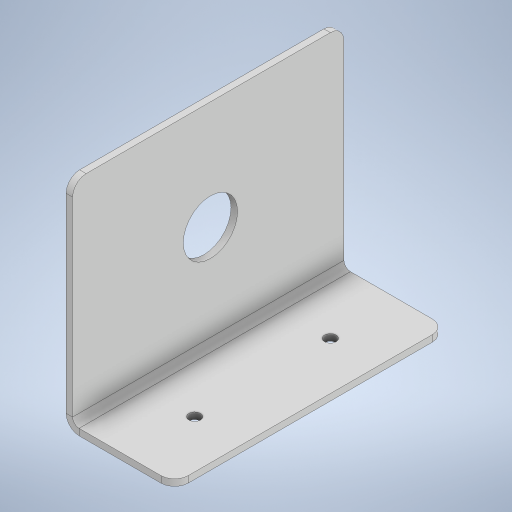
# Autodesk Inventor part: Bracket
Saved by Autodesk Inventor 2023 (Build 270158030, 158C)
## iProperties
Created: 2022-10-06
Part Number: Bracket
Material: Generic
Document SubType Name: Sheet Metal
Designer: cjj5381
Density: 1 g/cm^3
Sheet Metal Rule: Default
Appearance: Default
Author: cjj5381
Autodesk Inventor part; units mm, degrees
ref_plane "YZ Plane" through (0, 0, 0) normal (1, 0, 0) x (0, 1, 0)
ref_plane "XZ Plane" through (0, 0, 0) normal (0, 1, 0) x (-1, 0, 0)
ref_plane "XY Plane" through (0, 0, 0) normal (0, 0, 1) x (1, 0, 0)
sketch "Sketch1" plane through (0, 0, 0) normal (0, 1, 0) x (-1, 0, 0)
  line L0 (-25.4, 63.5) -> (25.4, 63.5)
  line L1 (25.4, 63.5) -> (25.4, -63.5)
  line L2 (25.4, -63.5) -> (-25.4, -63.5)
  line L3 (-25.4, -63.5) -> (-25.4, 63.5)
  line L4 (-25.4, 63.5) -> (25.4, -63.5) construction
  line L5 (25.4, 63.5) -> (-25.4, -63.5) construction
  point P0 (0, 0)
  dimension "d0" = 50.8
  dimension "d1" = 127
  measures "d0" distance of L1.end L2.end
  measures "d1" distance of L0.end L1.end
extrude "Plate1" add sketch "Sketch1" along normal blind 3.048
sketch "Sketch2" plane through (-22.352, 0, 63.5) normal (-1, 0, 0) x (0, -1, 0)
  line L0 (0, -127) -> (0, 0)
  line L1 (0, 0) -> (-101.6, 0)
  line L2 (-101.6, 0) -> (-101.6, -127)
  line L3 (-101.6, -127) -> (0, -127)
  constraints: 6 end point, 1 horizontal, 1 perpendicular, 1 vertical
edge flange "Flange1" height 101.6 angle 90 thickness 3.048 bend radius 3.048 thickness toward (-1, 0, 0) relief straight relief width 3.048 relief depth 1.524 edges at (-25.4, 3.048, 0) wall of the first edge with corners at (-22.352, 0, -63.5) (-22.352, 0, 63.5) (-22.352, 101.6, 63.5) (-22.352, 101.6, -63.5)
bend "Bend1"
corner "Corner1"
sketch "Sketch3" plane through (0, 3.048, 0) normal (0, 1, 0) x (1, 0, 0)
  line L0 (25.4, -63.5) -> (-19.304, -63.5) construction
  line L1 (3.048, -63.5) -> (3.048, 63.5) construction
  line L2 (-19.304, 63.5) -> (25.4, 63.5) construction
  point P0 (0, 0)
  point P1 (3.048, -31.75)
  point P2 (3.048, 31.75)
  dimension "d20" = 63.5
  dimension "d21" = 31.75
  constraints: 2 end point, 2 midpoint, 2 point on line, 1 vertical
  measures "d20" distance of point (3.048, 31.75) point (3.048, -31.75)
  measures "d21" vertical distance of point (3.048, 31.75) point (0, 0)
hole "Hole1" at (3.048, 3.048, 31.75) at (3.048, 3.048, -31.75) direction (0, -1, 0) diameter 5.5118 end through all clearance for "Hex Head Cap Screw ISO 24017" size "M5" standard "ISO"
fillet "Corner Round1" radius 6.35 4 edges at (-23.876, 101.6, 63.5) (25.4, 1.524, 63.5) (25.4, 1.524, -63.5) (-23.876, 101.6, -63.5)
sketch "Sketch4" plane through (-22.352, 6.096, 63.5) normal (1, 0, 0) x (0, 0, -1)
  line L0 (0, 0) -> (0, 89.154) construction
  line L1 (120.65, 95.504) -> (6.35, 95.504) construction
  point P0 (63.5, -6.096)
  point P1 (64.516, 44.704)
  dimension "d23" = 64.516
  dimension "d31" = 50.8
  measures "d23" distance from line of L0 point (64.516, 44.704)
  measures "d31" distance from line of L1 point (64.516, 44.704)
hole "Hole2" at (-22.352, 50.8, -1.016) direction (-1, 0, 0) diameter 25.4 end through all
equation "\"d21\" = 0.5 * d20"
equation "\"d18\" = Thickness"
equation "\"d2\" = Thickness"
equation "\"d3\" = BendReliefWidth"
equation "\"d4\" = BendReliefDepth"
equation "\"d5\" = MinimumRemnant"
equation "\"d6\" = TransitionRadius"
equation "\"d9\" = BendRadius"
equation "\"d10\" = CornerReliefSize"
equation "\"d11\" = GapSize"
equation "\"d12\" = JacobiRadiusSize"
equation "\"BendRadius\" = Thickness"
equation "\"BendReliefWidth\" = Thickness"
equation "\"BendReliefDepth\" = 0.5 * Thickness"
equation "\"CornerReliefSize\" = 4 * Thickness"
equation "\"MinimumRemnant\" = 2 * Thickness"
equation "\"TransitionRadius\" = BendRadius"
equation "\"JacobiRadiusSize\" = BendRadius"
equation "\"GapSize\" = Thickness"
equation "\"Thickness\" = 3.048"
body "Solid1"
